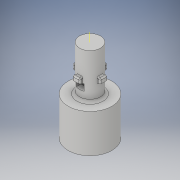
# Autodesk Inventor part: SoportePulgada
Saved by Autodesk Inventor 2019 (Build 230136000, 136)
## iProperties
Created: 2020-03-30
Part Number: SoportePulgada
Material: Generic
Document SubType Name: Modeling
Designer: Sergio
Density: 1 g/cm^3
Appearance: Default
Author: Sergio
Autodesk Inventor part; units mm, degrees
ref_plane "YZ Plane" through (0, 0, 0) normal (1, 0, 0) x (0, 1, 0)
ref_plane "XZ Plane" through (0, 0, 0) normal (0, 1, 0) x (-1, 0, 0)
ref_plane "XY Plane" through (0, 0, 0) normal (0, 0, 1) x (1, 0, 0)
sketch "Sketch1" plane through (0, 0, 0) normal (0, 1, 0) x (-1, 0, 0)
  circle A0 centre (0, 0) radius 8.225
  dimension "d0" = 16.45
  constraints: 1 centre point
  measures "d0" diameter of A0
extrude "Extrusion1" add sketch "Sketch1" along normal blind 35
sketch "Sketch2" plane through (0, 0, 0) normal (0, -1, 0) x (1, 0, 0)
  circle A0 centre (0, 0) radius 17.05
  dimension "d3" = 34.1
  constraints: 1 centre point, 1 coincident
  measures "d3" diameter of A0
extrude "Extrusion2" add sketch "Sketch2" along normal blind 30
sketch "Sketch3" plane through (0, 0, 0) normal (1, 0, 0) x (0, 1, 0)
  line L0 (-30, 17.05) -> (-30, -17.05) projected
  line L1 (7, 4) -> (-30, 4)
  line L2 (-30, 4) -> (-30, -4)
  line L3 (-30, -4) -> (7, -4)
  line L4 (0, 8.225) -> (35, 8.225) projected
  line L5 (0, -8.225) -> (35, -8.225) projected
  line L6 (12, 8.225) -> (7, 8.225)
  line L7 (7, -8.225) -> (12, -8.225)
  line L8 (12, -8.225) -> (12, 8.225)
  line L9 (7, 8.225) -> (7, 4)
  line L10 (7, -4) -> (7, -8.225)
  point P0 (0, 0)
  dimension "d7" = 4
  dimension "d8" = 4
  dimension "d12" = 5
  dimension "d13" = 37
  constraints: 16 end point, 4 parallel, 3 perpendicular, 3 point on line, 2 horizontal
  measures "d7" distance from line of L3 point (0, 0)
  measures "d8" distance from line of point (0, 0) L1
  measures "d12" distance between parallel lines of L10 L8
  measures "d13" distance between parallel lines of L0 L10
extrude "Extrusion3" cut sketch "Sketch3" along normal mid plane 6
sketch "Sketch4" plane through (0, 0, 0) normal (1, 0, 0) x (0, 1, 0)
  line L0 (12, -8.225) -> (12, -7.6584) projected
  line L1 (12, -8.225) -> (16.8057, -8.225)
  line L2 (16.8057, -8.225) -> (16.8057, -11.025)
  line L3 (16.8057, -11.025) -> (13.3057, -11.025)
  line L4 (-7, 0) -> (42, 0) projected
  line L5 (13.3057, -11.025) -> (12, -8.225)
  line L6 (12, -8.225) -> (12, -8.225)
  line L7 (0, -8.225) -> (35, -8.225) projected
  point P0 (0, 0)
  dimension "d14" = 3.5
  dimension "d15" = 2.8
  dimension "d20" = 65
  dimension "d21" = 0
  constraints: 10 end point, 1 collinear, 1 horizontal, 1 parallel, 1 perpendicular
  measures "d14" distance of L2.end L3.end
  measures "d15" distance of L1.end L2.end
  measures "d20" angle of L6 L5
  measures "d21" distance of L5.end L0.start
revolve "Revolution1" add sketch "Sketch4" angle 33 mid plane about axis through (0, -10, 0) along (0, 1, 0)
fillet "Fillet1" radius 1 1 edges at (0, 16.8057, -11.025)
fillet "Fillet3" radius 1 3 edges at (-2.5916, 16.8057, -8.7492) (-3.1313, 14.5557, -10.571) (-3.0481, 16.5128, -10.2902)
fillet "Fillet4" radius 1 3 edges at (3.1313, 14.5557, -10.571) (2.5916, 16.8057, -8.7492) (3.0481, 16.5128, -10.2902)
pattern_circular "Circular Pattern2" count 4 over 360 about axis through (0, -10, 0) along (0, 1, 0) of "Revolution1", "Fillet1", "Fillet3", "Fillet4"
fillet "Fillet5" radius 2 1 edges at (8.225, 0, 0)
body "Solid1"
